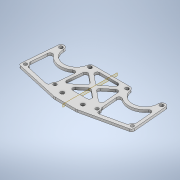
# Autodesk Inventor part: Knee_side_frame
Saved by Autodesk Inventor 2022.4 (Build 264492000, 492)
## iProperties
Created: 2021-09-05
Part Number: Knee_side_frame
Material: アルミニウム 2014-T4
Document SubType Name: Modeling
Designer: Masato Kubotera
Density: 2.8 g/cm^3
Appearance: 滑らか - 淡い灰色
Mass: 7.94371 g
Surface Area: 42.7962 cm^2
Volume: 2.83704 cm^3
Description: A2017 T2
Author: Masato Kubotera
Autodesk Inventor part; units mm, degrees
ref_plane "YZ Plane" through (0, 0, 0) normal (1, 0, 0) x (0, 1, 0)
ref_plane "XY Plane" through (0, 0, 0) normal (0, 0, 1) x (1, 0, 0)
sketch "スケッチ1" plane through (0, 0, 0) normal (0, 0, 1) x (1, 0, 0)
  line L0 (-32.0417, 43.3932) -> (10.7946, 47.1409) construction
  line L1 (10.7946, 47.1409) -> (13.5836, 15.2627) construction
  line L2 (13.5836, 15.2627) -> (-29.2527, 11.515) construction
  line L3 (-29.2527, 11.515) -> (-32.0417, 43.3932) construction
  line L4 (-32.0417, 43.3932) -> (13.5836, 15.2627) construction
  line L5 (10.7946, 47.1409) -> (-29.2527, 11.515) construction
  line L6 (-30.6472, 27.4541) -> (12.1891, 31.2018) construction
  line L7 (8.0239, 44.389) -> (-18.8733, 42.0358) construction
  line L8 (-18.8733, 42.0358) -> (-16.5201, 15.1385) construction
  line L9 (-16.5201, 15.1385) -> (10.3771, 17.4917) construction
  line L10 (10.3771, 17.4917) -> (8.0239, 44.389) construction
  line L11 (8.0239, 44.389) -> (-16.5201, 15.1385) construction
  line L12 (-18.8733, 42.0358) -> (10.3771, 17.4917) construction
  circle A0 centre (-18.6929, 28.5) radius 10.5 construction
  line L13 (-5.4247, 43.2124) -> (-3.0715, 16.3151) construction
  circle A1 centre (8.0239, 44.389) radius 1.35
  circle A2 centre (10.3771, 17.4917) radius 1.35
  arc A3 (-21.6497, 41.7929) -> (-18.8362, 39.249) centre (-18.8733, 42.0358) ccw
  arc A4 (-16.9674, 17.8894) -> (-18.8362, 39.249) centre (-18.6929, 28.5) ccw
  arc A5 (-16.9674, 17.8894) -> (-19.3071, 15.1385) centre (-16.5201, 15.1385) ccw
  line L14 (-21.6497, 41.7929) -> (-21.8676, 44.2834)
  circle A6 centre (13.3071, 8.5) radius 1.55
  circle A7 centre (13.3071, 8.5) radius 6 construction
  circle A8 centre (13.3071, 8.5) radius 4.6 construction
  line L15 (19.3071, 8.5) -> (19.3071, -8.5)
  line L16 (-19.3071, 15.1385) -> (-19.3071, -15.1385)
  line L17 (-19.3071, 0) -> (19.3071, 0) construction
  line L18 (-21.8676, 44.2834) -> (10.7946, 47.1409)
  line L19 (10.7946, 47.1409) -> (19.1618, 9.8123)
  arc A9 (19.3071, 8.5) -> (19.1618, 9.8123) centre (13.3071, 8.5) ccw
  circle A10 centre (-18.6929, -28.5) radius 10.5 construction
  circle A11 centre (8.0239, -44.389) radius 1.35
  circle A12 centre (10.3771, -17.4917) radius 1.35
  arc A13 (-18.8362, -39.249) -> (-21.6497, -41.7929) centre (-18.8733, -42.0358) ccw
  arc A14 (-18.8362, -39.249) -> (-16.9674, -17.8894) centre (-18.6929, -28.5) ccw
  arc A15 (-19.3071, -15.1385) -> (-16.9674, -17.8894) centre (-16.5201, -15.1385) ccw
  line L20 (-21.6497, -41.7929) -> (-21.8676, -44.2834)
  circle A16 centre (13.3071, -8.5) radius 1.55
  circle A17 centre (13.3071, -8.5) radius 6 construction
  line L21 (-21.8676, -44.2834) -> (10.7946, -47.1409)
  line L22 (10.7946, -47.1409) -> (19.1618, -9.8123)
  arc A18 (19.1618, -9.8123) -> (19.3071, -8.5) centre (13.3071, -8.5) ccw
  line L23 (-16.5201, 15.1385) -> (10.3771, -17.4917) construction
  line L24 (-16.5201, -15.1385) -> (10.3771, 17.4917) construction
  line L25 (10.3771, -17.4917) -> (-16.5201, -15.1385) construction
  line L26 (-16.8071, 13.1284) -> (-5.9853, 0)
  line L27 (-16.8071, 13.1284) -> (-16.8071, -13.1284)
  line L28 (-13.7422, 14.1268) -> (-4.0414, 2.3583)
  line L29 (-4.0414, 2.3583) -> (7.1674, 15.9561)
  line L30 (-13.7422, 14.1268) -> (7.1674, 15.9561)
  line L31 (-17.2694, 42.1761) -> (5.5335, 44.1711)
  arc A19 (-11.404, 16.8409) -> (-17.2694, 42.1761) centre (-18.6929, 28.5) ccw
  line L32 (-11.404, 16.8409) -> (8.1114, 18.5483)
  line L33 (8.8648, 42.0346) -> (14.0135, 19.0646)
  arc A20 (5.5335, 44.1711) -> (8.8648, 42.0346) centre (8.0239, 44.389) ccw
  line L34 (-16.8071, -13.1284) -> (-5.9853, 0)
  arc A21 (12.425, 18.9257) -> (8.1114, 18.5483) centre (10.3771, 17.4917) ccw
  line L35 (12.425, 18.9257) -> (14.0135, 19.0646)
  line L36 (7.3071, 11.4091) -> (7.3071, -11.4091)
  line L37 (7.3071, 11.4091) -> (-2.0974, 0)
  line L38 (7.3071, -11.4091) -> (-2.0974, 0)
  line L39 (-13.7422, -14.1268) -> (-4.0414, -2.3583)
  line L40 (-4.0414, -2.3583) -> (7.1674, -15.9561)
  line L41 (-13.7422, -14.1268) -> (7.1674, -15.9561)
  line L42 (-17.2694, -42.1761) -> (5.5335, -44.1711)
  arc A22 (-17.2694, -42.1761) -> (-11.404, -16.8409) centre (-18.6929, -28.5) ccw
  line L43 (-11.404, -16.8409) -> (8.1114, -18.5483)
  line L44 (8.8648, -42.0346) -> (14.0135, -19.0646)
  arc A23 (8.8648, -42.0346) -> (5.5335, -44.1711) centre (8.0239, -44.389) ccw
  arc A24 (8.1114, -18.5483) -> (12.425, -18.9257) centre (10.3771, -17.4917) ccw
  line L45 (12.425, -18.9257) -> (14.0135, -19.0646)
  arc A25 (-17.5285, 42.1534) -> (-20.2182, 41.9181) centre (-18.8733, 42.0358) ccw
  arc A26 (-20.1746, 41.42) -> (-17.4849, 41.6553) centre (-18.8297, 41.5377) ccw
  line L46 (-20.2182, 41.9181) -> (-20.1746, 41.42)
  line L47 (-17.4849, 41.6553) -> (-17.5285, 42.1534)
  arc A27 (-17.865, 15.0209) -> (-15.1752, 15.2562) centre (-16.5201, 15.1385) ccw
  arc A28 (-15.2188, 15.7543) -> (-17.9085, 15.519) centre (-16.5637, 15.6366) ccw
  line L48 (-17.865, 15.0209) -> (-17.9085, 15.519)
  line L49 (-15.2188, 15.7543) -> (-15.1752, 15.2562)
  arc A29 (-20.2182, -41.9181) -> (-17.5285, -42.1534) centre (-18.8733, -42.0358) ccw
  arc A30 (-17.4849, -41.6553) -> (-20.1746, -41.42) centre (-18.8297, -41.5377) ccw
  line L50 (-20.2182, -41.9181) -> (-20.1746, -41.42)
  arc A31 (-17.9085, -15.519) -> (-15.2188, -15.7543) centre (-16.5637, -15.6366) ccw
  line L51 (-15.2188, -15.7543) -> (-15.1752, -15.2562)
  arc A32 (-15.1752, -15.2562) -> (-17.865, -15.0209) centre (-16.5201, -15.1385) ccw
  line L52 (-17.865, -15.0209) -> (-17.9085, -15.519)
  line L53 (-17.4849, -41.6553) -> (-17.5285, -42.1534)
  point P0 (0, 0)
  point P1 (-9.2291, 29.328)
  point P2 (-4.2481, 29.7638)
  dimension "d21" = 43
  dimension "d22" = 32
  dimension "d23" = 27
  dimension "d24" = 27
  dimension "d27" = 21
  dimension "d28" = 9.5
  dimension "d31" = 3.1
  dimension "d34" = 12
  dimension "d39" = 8.5
  dimension "d40" = 9.2
  dimension "d41" = 32
  dimension "d43" = 5
  dimension "d45" = 17
  dimension "d46" = 20
  dimension "d47" = 57
  dimension "d53" = 3
  dimension "d54" = 1.5
  dimension "d55" = 2.5
  dimension "d56" = 2.5
  dimension "d57" = 2.5
  dimension "d58" = 2.5
  dimension "d59" = 1.25
  dimension "d60" = 3
  dimension "d62" = 3
  dimension "d63" = 2.5
  dimension "d64" = 3
  dimension "d65" = 1.5
  dimension "d67" = 2.7
  dimension "d68" = 1.35
  dimension "d70" = 0.5
  dimension "d71" = 0.25
  constraints: 108 end point, 51 symmetric about line, 46 point on circle, 32 centre point, 15 parallel, 12 midpoint, 11 coincident, 10 tangent, 6 point on line, 4 perpendicular, 4 vertical, 1 collinear, 23 other
  measures "d21" distance of L1.end L2.end
  measures "d22" distance of L0.end L1.end
  measures "d23" distance of L9.end L8.end
  measures "d24" distance of L8.end L7.end
  measures "d27" diameter of A0
  measures "d28" distance of point (-9.229, 29.328) A0.centre
  measures "d31" diameter of A6
  measures "d34" diameter of A7
  measures "d39" distance from line of L8 point (-9.229, 29.328)
  measures "d40" diameter of A8
  measures "d41" horizontal distance of A6.centre A0.centre
  measures "d43" angle of L17 L2
  measures "d45" distance of A16.centre A6.centre
  measures "d46" vertical distance of A9.centre A0.centre
  measures "d47" distance of A14.centre A0.centre
  measures "d53" distance between parallel lines of L26 L28
  measures "d54" distance between parallel lines of L23 L26
  measures "d55" distance between parallel lines of L16 L27
  measures "d56" radius of A20
  measures "d57" distance from line of L31.end L18
  measures "d58" distance between parallel lines of L32 L30
  measures "d59" distance between parallel lines of L30 L9
  measures "d60" radial gap between concentric circles of A19 A4
  measures "d62" distance between parallel lines of L19 L33
  measures "d63" radius of A21
  measures "d64" distance between parallel lines of L37 L29
  measures "d65" distance between parallel lines of L37 L24
  measures "d67" diameter of A1
  measures "d68" radius of A25
  measures "d70" distance of L47.start L47.end
  measures "d71" radial gap between concentric circles of A0 A4
extrude "押し出し1" add sketch "スケッチ1" along normal blind 2
fillet "フィレット1" radius 2 4 edges at (-21.8676, 44.2834, 1) (-21.8676, -44.2834, 1) (10.7946, -47.1409, 1) (10.7946, 47.1409, 1)
fillet "フィレット2" radius 2 26 edges at (-17.2694, 42.1761, 1) (-11.404, 16.8409, 1) (14.0135, 19.0646, 1) (12.425, 18.9257, 1) (8.1114, 18.5483, 1) (5.5335, 44.1711, 1) (8.8648, 42.0346, 1) (-13.7422, 14.1268, 1) (-16.8071, 13.1284, 1) (-16.8071, -13.1284, 1) (-5.9853, 0, 1) (-4.0414, 2.3583, 1) (-2.0974, 0, 1) (-13.7422, -14.1268, 1) (7.1674, -15.9561, 1) (7.3071, -11.4091, 1) (7.3071, 11.4091, 1) (7.1674, 15.9561, 1) (-11.404, -16.8409, 1) (12.425, -18.9257, 1) (14.0135, -19.0646, 1) (8.1114, -18.5483, 1) (-17.2694, -42.1761, 1) (8.8648, -42.0346, 1) (5.5335, -44.1711, 1) (-4.0414, -2.3583, 1)
